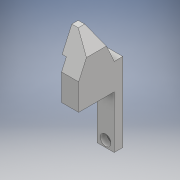
# Autodesk Inventor part: armmodulepart2
Saved by Autodesk Inventor 2018.3 (Build 223284000, 284)
## iProperties
Created: 2019-11-02
Part Number: armmodulepart2
Material: 一般
Document SubType Name: Modeling
Designer: Eiji Nishizawa
Density: 1 g/cm^3
Appearance: 既定
Author: Eiji Nishizawa
Autodesk Inventor part; units mm, degrees
ref_plane "YZ Plane" through (0, 0, 0) normal (1, 0, 0) x (0, 1, 0)
ref_plane "XZ Plane" through (0, 0, 0) normal (0, 1, 0) x (-1, 0, 0)
ref_plane "XY Plane" through (0, 0, 0) normal (0, 0, 1) x (1, 0, 0)
sketch "スケッチ1" plane through (0, 0, 0) normal (0, 1, 0) x (-1, 0, 0)
  line L0 (4.4873, 36.645) -> (-3.5127, 36.645)
  line L1 (-3.5127, 36.645) -> (-3.5127, -15.255)
  line L2 (-3.5127, -15.255) -> (4.4873, -15.255)
  line L3 (4.4873, -15.255) -> (4.4873, 36.645)
  circle A0 centre (0.4873, -12.255) radius 2.5
  line L4 (4.4873, 36.645) -> (9.3325, 36.645)
  line L5 (9.3325, 36.645) -> (9.3325, 26.645)
  line L6 (9.3325, 26.645) -> (4.4873, 26.645)
  line L7 (4.4873, 26.645) -> (4.4873, 36.645)
  point P0 (0, 0)
  dimension "d0" = 5
  dimension "d1" = 3
  dimension "d2" = 4
  dimension "d3" = 4
  dimension "d4" = 46.4
  dimension "d5" = 10
  constraints: 16 end point, 4 parallel, 2 horizontal, 2 perpendicular, 1 centre point
  measures "d0" diameter of A0
  measures "d1" distance from line of L2 A0.centre
  measures "d2" distance from line of L3 A0.centre
  measures "d3" distance from line of L1 A0.centre
  measures "d4" distance edge to line of A0 L0
  measures "d5" distance between parallel lines of L4 L6
extrude "押し出し1" add sketch "スケッチ1" against normal blind 3 contours L3 L2 L1 L0
sketch "スケッチ2" plane through (0, 0, 0) normal (0, 1, 0) x (1, 0, 0)
  line L0 (3.5127, -36.645) -> (-4.4873, -36.645) projected
  line L1 (3.5127, 15.255) -> (3.5127, -36.645) projected
  line L2 (-4.4873, -36.645) -> (3.5127, -36.645)
  line L3 (3.5127, -36.645) -> (3.5127, 15.255)
  line L4 (3.5127, 15.255) -> (-4.4873, 15.255)
  line L5 (-4.4873, 15.255) -> (-4.4873, -36.645)
  circle A0 centre (-0.4873, 12.255) radius 1.5
  circle A1 centre (-0.4873, 12.255) radius 2.5 projected
  point P0 (0, 0)
  dimension "d8" = 3
  constraints: 8 end point, 2 parallel, 1 centre point, 1 concentric, 1 horizontal, 1 perpendicular
  measures "d8" diameter of A0
extrude "押し出し2" add sketch "スケッチ2" along normal blind 1 contours L0 L5 L4 L1 | A1
sketch "スケッチ3" plane through (0, -3, 0) normal (0, -1, 0) x (1, 0, 0)
  line L0 (-4.4873, 36.645) -> (-4.4873, -15.255) projected
  line L1 (-4.4873, 36.645) -> (-6.4873, 36.645)
  line L2 (-6.4873, 36.645) -> (-6.4873, 26.645)
  line L3 (-6.4873, 26.645) -> (-4.4873, 26.645)
  line L4 (-4.4873, 26.645) -> (-4.4873, 36.645)
  line L5 (-4.4873, 36.645) -> (3.5127, 36.645)
  line L6 (3.5127, 36.645) -> (3.5127, 9.2999)
  line L7 (3.5127, 9.2999) -> (-4.4873, 9.2999)
  line L8 (-4.4873, 9.2999) -> (-4.4873, 36.645)
  line L9 (3.5127, -15.255) -> (3.5127, 36.645) projected
  point P0 (0, 0)
  dimension "d11" = 10
  dimension "d12" = 0
  dimension "d24" = 2
  constraints: 16 end point, 4 parallel, 2 horizontal, 2 perpendicular
  measures "d11" distance of L1.end L2.end
  measures "d12" distance between parallel lines of L9 L6
  measures "d24" distance of L0.start L1.end
extrude "押し出し3" add sketch "スケッチ3" along normal blind 16.6
chamfer "面取り1" distance 7 angle 45 1 edges at (3.5127, -9.3, 36.645)
chamfer "面取り3" distance 15 distance2 6.8 1 edges at (-4.9873, -19.6, 36.645) measured on face at (0.846, -19.6, 21.8633)
sketch "スケッチ4" plane through (0, 1, 0) normal (0, 1, 0) x (1, 0, 0)
  line L0 (-4.4873, -36.645) -> (-6.4873, -36.645) projected
  line L1 (3.5127, -9.2999) -> (-4.4873, -9.2999) projected
  line L2 (-6.4873, -36.645) -> (3.5127, -36.645)
  line L3 (3.5127, -36.645) -> (3.5127, -9.2999)
  line L4 (3.5127, -9.2999) -> (-6.4873, -9.2999)
  line L5 (-6.4873, -9.2999) -> (-6.4873, -36.645)
  point P0 (0, 0)
  constraints: 8 end point, 2 parallel, 1 collinear, 1 horizontal, 1 perpendicular
extrude "押し出し4" cut sketch "スケッチ4" against normal blind 4
chamfer "面取り4" distance 6.8 distance2 15 1 edges at (-4.9873, -3, 36.645) measured on face at (-4.4873, -9.5333, 36.645)
sketch "スケッチ5" plane through (0, -3, 0) normal (0, 1, 0) x (1, 0, 0)
  line L0 (3.5127, -21.645) -> (-4.4873, -21.645) projected
  line L1 (-4.4873, -9.2999) -> (-4.4873, 15.255) projected
  line L2 (3.5127, -21.645) -> (-4.4873, -21.645)
  line L3 (-4.4873, -21.645) -> (-4.4873, -9.2999)
  line L4 (-4.4873, -9.2999) -> (3.5127, -9.2999)
  line L5 (3.5127, -9.2999) -> (3.5127, -21.645)
  point P0 (0, 0)
  constraints: 8 end point, 2 parallel, 1 horizontal, 1 perpendicular
extrude "押し出し5" add sketch "スケッチ5" along normal blind 4
